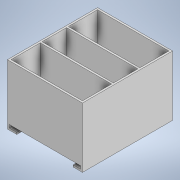
# Autodesk Inventor part: BeadCompartments_1
Saved by Autodesk Inventor 2020 (Build 240168000, 168)
## iProperties
Created: 2021-12-08
Part Number: BeadCompartments_1
Material: Generic
Document SubType Name: Modeling
Designer: danie
Density: 1 g/cm^3
Appearance: Default
Author: danie
Autodesk Inventor part; units mm, degrees
ref_plane "YZ Plane" through (0, 0, 0) normal (1, 0, 0) x (0, 1, 0)
ref_plane "XZ Plane" through (0, 0, 0) normal (0, 1, 0) x (-1, 0, 0)
ref_plane "XY Plane" through (0, 0, 0) normal (0, 0, 1) x (1, 0, 0)
sketch "Sketch1" plane through (0, 0, 0) normal (0, 1, 0) x (-1, 0, 0)
  line L0 (0, 0) -> (-3.175, 0)
  line L1 (-3.175, 0) -> (-3.175, 152.4)
  line L2 (-3.175, 152.4) -> (0, 152.4)
  line L3 (0, 152.4) -> (0, 0)
  dimension "d0" = 3.175
  dimension "d1" = 152.4
  constraints: 8 end point, 2 parallel, 1 horizontal, 1 perpendicular
  measures "d0" distance of L1.end L2.end
  measures "d1" distance of L0.end L1.end
extrude "Extrusion1" add sketch "Sketch1" along normal blind 50.8
sketch "Sketch2" plane through (0, 0, 0) normal (0, -1, 0) x (1, 0, 0)
  line L0 (0, 0) -> (127, 0) construction
  line L1 (0, 0) -> (127, 0) construction
  line L2 (127, 0) -> (123.825, 0)
  line L3 (123.825, 0) -> (123.825, 152.4)
  line L4 (123.825, 152.4) -> (127, 152.4)
  line L5 (127, 152.4) -> (127, 0)
  dimension "d4" = 127
  dimension "d5" = 0
  dimension "d6" = 3.175
  dimension "d7" = 152.4
  constraints: 12 end point, 3 horizontal, 2 parallel, 1 collinear, 1 perpendicular
  measures "d4" distance of L0.start L0.end
  measures "d5" distance between parallel lines of L0 L1
  measures "d6" distance of L3.end L4.end
  measures "d7" distance of L2.end L3.end
extrude "Extrusion2" add sketch "Sketch2" against normal blind 50.8
sketch "Sketch3" plane through (0, 0, 152.4) normal (0, 0, 1) x (1, 0, 0)
  line L0 (3.175, 0) -> (3.175, 50.8) projected
  line L1 (3.175, 0) -> (15.875, 0)
  line L2 (15.875, 0) -> (15.875, 3.175)
  line L3 (15.875, 3.175) -> (3.175, 3.175)
  line L4 (3.175, 3.175) -> (3.175, 0)
  point P0 (0, 0)
  point P1 (3.175, 3.175)
  dimension "d10" = 12.7
  dimension "d11" = 3.175
  constraints: 8 end point, 2 parallel, 1 horizontal, 1 perpendicular
  measures "d10" distance of L3.end L2.end
  measures "d11" distance of L2.end L1.end
extrude "Extrusion3" add sketch "Sketch3" against normal blind 152.4
sketch "Sketch4" plane through (123.825, 0, 152.4) normal (0, 0, 1) x (1, 0, 0)
  line L0 (0, 0) -> (0, 50.8) projected
  line L1 (0, 0) -> (-12.7, 0)
  line L2 (-12.7, 0) -> (-12.7, 3.175)
  line L3 (-12.7, 3.175) -> (0, 3.175)
  line L4 (0, 3.175) -> (0, 0)
  point P0 (-123.825, 0)
  dimension "d14" = 12.7
  dimension "d15" = 3.175
  constraints: 8 end point, 2 parallel, 1 horizontal, 1 perpendicular
  measures "d14" distance of L2.end L3.end
  measures "d15" distance of L1.end L2.end
extrude "Extrusion4" add sketch "Sketch4" against normal blind 152.4
sketch "Sketch5" plane through (0, 50.8, 152.4) normal (0, 0, 1) x (1, 0, 0)
  line L0 (15.875, -47.625) -> (3.175, -47.625) construction
  line L1 (3.175, -47.625) -> (3.175, -42.545) construction
  line L2 (3.175, -47.625) -> (3.175, 0) construction
  line L3 (127, 0) -> (123.825, 0) projected
  line L4 (3.175, -42.545) -> (123.825, -42.545)
  line L5 (123.825, -42.545) -> (123.825, 0)
  line L6 (123.825, 0) -> (3.175, 0)
  line L7 (3.175, 0) -> (3.175, -42.545)
  point P0 (0, -50.8)
  dimension "d18" = 5.08
  constraints: 10 end point, 2 parallel, 1 horizontal, 1 perpendicular, 1 point on line
  measures "d18" distance of L0.end L1.end
extrude "Extrusion5" add sketch "Sketch5" against normal blind 3.175
sketch "Sketch6" plane through (127, 50.8, 0) normal (0, 0, -1) x (-1, 0, 0)
  line L0 (0, 0) -> (3.175, 0) projected
  line L1 (123.825, -42.545) -> (3.175, -42.545) projected
  line L2 (3.175, 0) -> (123.825, 0)
  line L3 (123.825, 0) -> (123.825, -42.545)
  line L4 (123.825, -42.545) -> (3.175, -42.545)
  line L5 (3.175, -42.545) -> (3.175, 0)
  point P0 (127, -50.8)
  constraints: 8 end point, 2 parallel, 1 horizontal, 1 perpendicular
extrude "Extrusion6" add sketch "Sketch6" against normal blind 3.175
sketch "Sketch8" plane through (3.175, 3.175, 152.4) normal (1, 0, 0) x (0, 0, -1)
  line L0 (3.175, 47.625) -> (53.975, 47.625) construction
  line L1 (3.175, 47.625) -> (149.225, 47.625) construction
  line L2 (3.175, 47.625) -> (53.975, 47.625) construction
  line L3 (152.4, -3.175) -> (0, -3.175) construction
  line L4 (53.975, 47.625) -> (101.6, 47.625) construction
  line L5 (53.975, 0) -> (53.975, 5.08) construction
  line L6 (53.975, 47.625) -> (53.975, 5.08) construction
  line L7 (52.3875, 47.625) -> (55.5625, 47.625)
  line L8 (55.5625, 47.625) -> (55.5625, 5.08)
  line L9 (55.5625, 5.08) -> (52.3875, 5.08)
  line L10 (52.3875, 5.08) -> (52.3875, 47.625)
  line L11 (52.3875, 47.625) -> (55.5625, 5.08) construction
  line L12 (55.5625, 47.625) -> (52.3875, 5.08) construction
  point P0 (53.975, 26.3525)
  dimension "d26" = 50.8
  dimension "d27" = 0
  dimension "d28" = 47.625
  dimension "d30" = 5.08
  dimension "d32" = 3.175
  constraints: 22 end point, 3 horizontal, 3 midpoint, 2 collinear, 2 parallel, 1 perpendicular, 1 vertical
  measures "d26" distance of L0.start L0.end
  measures "d27" distance between parallel lines of L0 L2
  measures "d28" distance of L2.end L5.start
  measures "d30" distance of L5.start L5.end
  measures "d32" distance of L8.end L9.end
extrude "Extrusion7" add sketch "Sketch8" along normal up to next
sketch "Sketch9" plane through (3.175, 3.175, 152.4) normal (1, 0, 0) x (0, 0, -1)
  line L0 (149.225, 5.08) -> (149.225, 47.625) construction
  line L1 (149.225, 47.625) -> (98.425, 47.625) construction
  line L2 (55.5625, 47.625) -> (149.225, 47.625) construction
  line L3 (98.425, 47.625) -> (146.05, 47.625) construction
  line L4 (98.425, 0) -> (98.425, 5.08) construction
  line L5 (98.425, 47.625) -> (98.425, 5.08) construction
  line L6 (96.8375, 47.625) -> (100.0125, 47.625)
  line L7 (100.0125, 47.625) -> (100.0125, 5.08)
  line L8 (100.0125, 5.08) -> (96.8375, 5.08)
  line L9 (96.8375, 5.08) -> (96.8375, 47.625)
  line L10 (96.8375, 47.625) -> (100.0125, 5.08) construction
  line L11 (100.0125, 47.625) -> (96.8375, 5.08) construction
  point P0 (152.4, -3.175)
  point P1 (98.425, 26.3525)
  dimension "d35" = 50.8
  dimension "d36" = 47.625
  dimension "d38" = 5.08
  dimension "d40" = 3.175
  dimension "d41" = 42.545
  constraints: 20 end point, 3 midpoint, 2 horizontal, 2 parallel, 2 perpendicular, 1 point on line
  measures "d35" distance of L0.end L1.end
  measures "d36" distance of L1.end L4.start
  measures "d38" distance of L4.start L4.end
  measures "d40" distance of L7.end L8.end
  measures "d41" distance of L6.end L7.end
extrude "Extrusion8" add sketch "Sketch9" along normal up to next
sketch "Sketch10" plane through (0, 50.8, 0) normal (0, 1, 0) x (1, 0, 0)
  line L0 (3.175, -55.5625) -> (123.825, -55.5625) construction
  line L1 (123.825, -55.5625) -> (127, -55.5625) construction
  line L2 (127, 0) -> (127, -152.4) construction
  line L3 (3.175, -100.0125) -> (123.825, -100.0125) construction
  line L4 (3.175, -100.0125) -> (0, -100.0125) construction
  line L5 (127, 0) -> (0, 0) projected
  line L6 (0, 0) -> (127, 0)
  line L7 (127, 0) -> (127, -55.5625)
  line L8 (127, -55.5625) -> (0, -55.5625)
  line L9 (0, -55.5625) -> (0, 0)
  line L10 (3.175, -3.175) -> (123.825, -3.175)
  line L11 (123.825, -3.175) -> (123.825, -52.3875)
  line L12 (123.825, -52.3875) -> (3.175, -52.3875)
  line L13 (3.175, -52.3875) -> (3.175, -3.175)
  line L14 (0, -100.0125) -> (127, -100.0125)
  line L15 (127, -100.0125) -> (127, -52.3875)
  line L16 (127, -52.3875) -> (0, -52.3875)
  line L17 (0, -52.3875) -> (0, -100.0125)
  line L18 (3.175, -96.8375) -> (123.825, -96.8375)
  line L19 (123.825, -96.8375) -> (123.825, -55.5625)
  line L20 (123.825, -55.5625) -> (3.175, -55.5625)
  line L21 (3.175, -55.5625) -> (3.175, -96.8375)
  line L22 (0, 0) -> (0, -152.4) projected
  line L23 (0, -152.4) -> (127, -152.4)
  line L24 (127, -152.4) -> (127, -96.8375)
  line L25 (127, -96.8375) -> (0, -96.8375)
  line L26 (0, -96.8375) -> (0, -152.4)
  line L27 (123.825, -149.225) -> (3.175, -149.225)
  line L28 (3.175, -149.225) -> (3.175, -100.0125)
  line L29 (3.175, -100.0125) -> (123.825, -100.0125)
  line L30 (123.825, -100.0125) -> (123.825, -149.225)
  point P0 (3.175, -55.5625)
  dimension "d44" = 3.175
  dimension "d45" = 3.175
  dimension "d46" = 3.175
  constraints: 52 end point, 12 parallel, 6 perpendicular, 5 horizontal, 3 point on line, 9 other
  measures "d44" distance between parallel lines of L9 L13
  measures "d45" distance between parallel lines of L17 L21
  measures "d46" distance between parallel lines of L23 L27
extrude "Extrusion9" add sketch "Sketch10" along normal blind 50.8 contours L7 L16 L11 L10 L13 L9 L5 | L7 L8 L9 L16 L12 | L15 L25 L19 L8 | L8 L21 L25 L17 | L15 L14 L17 L25 L18 | L24 L23 L22 L14 L28 L27 L30
body "Solid1"
